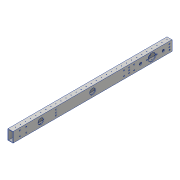
# Autodesk Inventor part: Drive Frame Rail
Saved by Autodesk Inventor 2018 (Build 220112000, 112)
## iProperties
Created: 2018-01-08
Part Number: Drive Frame Rail
Material: Aluminum 6061
Document SubType Name: Modeling
Designer: dsayers
Density: 2.7 g/cm^3
Appearance: Aluminum - Flat
Mass: 735.174 g
Surface Area: 2200.06 cm^2
Volume: 272.287 cm^3
Author: dsayers
Autodesk Inventor part; units mm, degrees
ref_plane "YZ Plane" through (0, 0, 0) normal (1, 0, 0) x (0, 1, 0)
ref_plane "XZ Plane" through (0, 0, 0) normal (0, 1, 0) x (-1, 0, 0)
ref_plane "XY Plane" through (0, 0, 0) normal (0, 0, 1) x (1, 0, 0)
sketch "Sketch1" plane through (0, 0, 0) normal (0, 0, 1) x (1, 0, 0)
  line L0 (0, 0) -> (25.4, 0)
  line L1 (25.4, 0) -> (25.4, 50.8)
  line L2 (25.4, 50.8) -> (0, 50.8)
  line L3 (0, 50.8) -> (0, 0)
  dimension "d0" = 25.4
  dimension "d1" = 50.8
  constraints: 8 end point, 2 parallel, 1 horizontal, 1 perpendicular
  measures "d0" distance of L1.end L2.end
  measures "d1" distance of L0.end L1.end
extrude "Extrusion1" add sketch "Sketch1" along normal blind 800.1
shell "Shell1" thickness 2.54 removed faces 2 at (8.4667, 33.8667, 0) at (8.4667, 33.8667, 800.1)
sketch "Sketch2" plane through (0, 50.8, 0) normal (0, 1, 0) x (1, 0, 0)
  line L0 (25.4, 0) -> (0, 0) projected
  line L1 (0, 0) -> (0, -800.1) projected
  point P0 (12.7, -12.7)
  point P1 (12.7, -38.1)
  point P2 (12.7, -63.5)
  point P3 (12.7, -88.9)
  point P4 (12.7, -114.3)
  point P5 (12.7, -139.7)
  point P6 (12.7, -165.1)
  point P7 (12.7, -190.5)
  point P8 (12.7, -215.9)
  point P9 (12.7, -241.3)
  point P10 (12.7, -266.7)
  point P11 (12.7, -292.1)
  point P12 (12.7, -317.5)
  point P13 (12.7, -342.9)
  point P14 (12.7, -368.3)
  point P15 (12.7, -393.7)
  point P16 (12.7, -419.1)
  point P17 (12.7, -444.5)
  point P18 (12.7, -469.9)
  point P19 (12.7, -495.3)
  point P20 (12.7, -520.7)
  point P21 (12.7, -546.1)
  point P22 (12.7, -571.5)
  point P23 (12.7, -596.9)
  point P24 (12.7, -622.3)
  point P25 (12.7, -647.7)
  point P26 (12.7, -673.1)
  point P27 (12.7, -698.5)
  point P28 (12.7, -723.9)
  point P29 (12.7, -749.3)
  point P30 (12.7, -774.7)
  dimension "d5" = 12.7
  dimension "d6" = 12.7
  dimension "d9" = 25.4
  constraints: 1 vertical, 30 other
  measures "d5" distance from line of L0 point (12.7, -12.7)
  measures "d6" distance from line of L1 point (12.7, -12.7)
  measures "d9" distance of point (12.7, -12.7) point (12.7, -38.1)
hole "Hole1" at (12.7, 50.8, 12.7) at (12.7, 50.8, 38.1) at (12.7, 50.8, 63.5) at (12.7, 50.8, 88.9) at (12.7, 50.8, 114.3) at (12.7, 50.8, 139.7) at (12.7, 50.8, 165.1) at (12.7, 50.8, 190.5) at (12.7, 50.8, 215.9) at (12.7, 50.8, 241.3) at (12.7, 50.8, 266.7) at (12.7, 50.8, 292.1) at (12.7, 50.8, 317.5) at (12.7, 50.8, 342.9) at (12.7, 50.8, 368.3) at (12.7, 50.8, 393.7) at (12.7, 50.8, 419.1) at (12.7, 50.8, 444.5) at (12.7, 50.8, 469.9) at (12.7, 50.8, 495.3) at (12.7, 50.8, 520.7) at (12.7, 50.8, 546.1) at (12.7, 50.8, 571.5) at (12.7, 50.8, 596.9) at (12.7, 50.8, 622.3) at (12.7, 50.8, 647.7) at (12.7, 50.8, 673.1) at (12.7, 50.8, 698.5) at (12.7, 50.8, 723.9) at (12.7, 50.8, 749.3) at (12.7, 50.8, 774.7) direction (0, -1, 0) diameter 2.54 depth 50.8 tip angle 118
sketch "Sketch3" plane through (25.4, 0, 0) normal (1, 0, 0) x (0, 0, -1)
  line L0 (0, 0) -> (0, 50.8) projected
  line L1 (0, 50.8) -> (-800.1, 50.8) projected
  point P0 (-101.6, 25.4)
  dimension "d21" = 101.6
  dimension "d22" = 25.4
  measures "d21" distance from line of L0 point (-101.6, 25.4)
  measures "d22" distance from line of L1 point (-101.6, 25.4)
hole "Hole2" at (25.4, 25.4, 101.6) direction (-1, 0, 0) diameter 38.1 depth 25.4 tip angle 118
sketch "Sketch4" plane through (25.4, 0, 0) normal (1, 0, 0) x (0, 0, -1)
  circle A0 centre (-101.6, 25.4) radius 19.05 projected
  line L0 (0, 0) -> (0, 50.8) projected
  line L1 (0, 50.8) -> (-800.1, 50.8) projected
  line L2 (-800.1, 0) -> (-800.1, 50.8) projected
  line L3 (0, 0) -> (-800.1, 0) projected
  point P0 (0, 0)
  point P1 (-125.4125, 25.4)
  point P2 (-77.7875, 25.4)
  dimension "d30" = 23.8125
  dimension "d31" = 23.8125
  dimension "d32" = 25.4
  dimension "d33" = 25.4
  measures "d30" distance of A0.centre point (-77.788, 25.4)
  measures "d31" distance of point (-125.412, 25.4) A0.centre
  measures "d32" distance from line of point (-77.788, 25.4) L1
  measures "d33" distance from line of L1 point (-125.412, 25.4)
hole "Hole3" at (25.4, 25.4, 125.4125) at (25.4, 25.4, 77.7875) direction (-1, 0, 0) diameter 5.6134 depth 25.4 tip angle 118 clearance for "Flat Head Machine Screw (82)" size "#10" standard "Ansi Unified Screw Threads"
sketch "Sketch5" plane through (25.4, 0, 0) normal (1, 0, 0) x (0, 0, -1)
  circle A0 centre (-44.45, 25.4) radius 8.0391 projected
  circle A1 centre (-158.75, 25.4) radius 9.5885 projected
  point P0 (0, 0)
  point P1 (26.2069, 26.9781)
  constraints: 2 coincident
hole "Hole4" at (25.4, 25.4, 158.75) at (25.4, 25.4, 44.45) at (25.4, 26.9781, -26.2069) direction (-1, 0, 0) diameter 12.7 depth 25.4 tip angle 118
sketch "Sketch6" plane through (0, 0, 0) normal (-1, 0, 0) x (0, 0, 1)
  line L0 (0, 50.8) -> (800.1, 50.8) projected
  line L1 (0, 50.8) -> (0, 0) projected
  line L2 (800.1, 50.8) -> (800.1, 0) projected
  point P0 (400.05, 25.4)
  point P1 (660.4, 25.4)
  dimension "d48" = 25.4
  dimension "d49" = 25.4
  dimension "d50" = 400.05
  dimension "d51" = 400.05
  dimension "d52" = 139.7
  measures "d48" distance from line of L0 point (660.4, 25.4)
  measures "d49" distance from line of L0 point (400.05, 25.4)
  measures "d50" distance from line of L1 point (400.05, 25.4)
  measures "d51" distance from line of L2 point (400.05, 25.4)
  measures "d52" distance from line of L2 point (660.4, 25.4)
hole "Hole5" at (0, 25.4, 400.05) at (0, 25.4, 660.4) direction (1, 0, 0) diameter 28.575 depth 25.4 tip angle 118
sketch "Sketch7" plane through (0, 0, 0) normal (-1, 0, 0) x (0, 0, 1)
  line L0 (723.9, 0) -> (723.9, 609.6)
  line L1 (774.7, 0) -> (774.7, 609.6)
  line L2 (0, 50.8) -> (800.1, 50.8) projected
  line L3 (0, 0) -> (800.1, 0) projected
  point P0 (733.425, 38.1)
  point P1 (765.175, 12.7)
  point P2 (733.425, 12.7)
  point P3 (765.175, 38.1)
  dimension "d60" = 9.525
  dimension "d61" = 9.525
  dimension "d62" = 12.7
  dimension "d63" = 12.7
  dimension "d64" = 12.7
  dimension "d65" = 12.7
  dimension "d66" = 9.525
  dimension "d67" = 9.525
  constraints: 4 end point, 2 vertical, 4 other
  measures "d60" distance from line of L1 point (765.175, 38.1)
  measures "d61" distance from line of L1 point (765.175, 12.7)
  measures "d62" distance from line of L2 point (765.175, 38.1)
  measures "d63" distance from line of L3 point (765.175, 12.7)
  measures "d64" distance from line of L3 point (733.425, 12.7)
  measures "d65" distance from line of L2 point (733.425, 38.1)
  measures "d66" distance from line of L0 point (733.425, 38.1)
  measures "d67" distance from line of L0 point (733.425, 12.7)
hole "Hole6" at (0, 38.1, 733.425) at (0, 12.7, 765.175) at (0, 12.7, 733.425) at (0, 38.1, 765.175) direction (1, 0, 0) diameter 5.6134 depth 25.4 tip angle 118 clearance for "Flat Head Machine Screw (82)" size "#10" standard "Ansi Unified Screw Threads"
sketch "Sketch8" plane through (25.4, 0, 0) normal (1, 0, 0) x (0, 0, -1)
  line L0 (-596.9, 50.8) -> (-596.9, 0) projected
  line L1 (-571.5, 0) -> (-571.5, 50.8) projected
  line L2 (-228.6, 50.8) -> (-228.6, 0) projected
  line L3 (-203.2, 0) -> (-203.2, 50.8) projected
  line L4 (0, 2.54) -> (0, 48.26) projected
  line L5 (-25.4, 50.8) -> (-25.4, 0) projected
  line L6 (0, 0) -> (0, 50.8) projected
  line L7 (0, 0) -> (-800.1, 0) projected
  line L8 (0, 50.8) -> (-800.1, 50.8) projected
  point P0 (-584.2, 38.1)
  point P1 (-584.2, 12.7)
  point P2 (-215.9, 38.1)
  point P3 (-215.9, 12.7)
  point P4 (-12.7, 38.1)
  point P5 (-12.7, 12.7)
  dimension "d75" = 12.7
  dimension "d76" = 12.7
  dimension "d77" = 12.7
  dimension "d78" = 12.7
  dimension "d79" = 12.7
  dimension "d80" = 12.7
  dimension "d81" = 12.7
  dimension "d82" = 12.7
  dimension "d83" = 12.7
  dimension "d84" = 12.7
  dimension "d85" = 12.7
  dimension "d86" = 12.7
  measures "d75" distance from line of point (-12.7, 38.1) L6
  measures "d76" distance from line of L6 point (-12.7, 12.7)
  measures "d77" distance from line of L7 point (-12.7, 12.7)
  measures "d78" distance from line of point (-12.7, 38.1) L8
  measures "d79" distance from line of L3 point (-215.9, 38.1)
  measures "d80" distance from line of L3 point (-215.9, 12.7)
  measures "d81" distance from line of point (-215.9, 12.7) L7
  measures "d82" distance from line of L8 point (-215.9, 38.1)
  measures "d83" distance from line of L1 point (-584.2, 38.1)
  measures "d84" distance from line of L1 point (-584.2, 12.7)
  measures "d85" distance from line of L8 point (-584.2, 38.1)
  measures "d86" distance from line of L7 point (-584.2, 12.7)
hole "Hole7" at (25.4, 38.1, 584.2) at (25.4, 12.7, 584.2) at (25.4, 38.1, 215.9) at (25.4, 12.7, 215.9) at (25.4, 38.1, 12.7) at (25.4, 12.7, 12.7) direction (-1, 0, 0) diameter 5.6134 depth 25.4 tip angle 118 clearance for "Flat Head Machine Screw (82)" size "#10" standard "Ansi Unified Screw Threads"
sketch "Sketch9" plane through (25.4, 0, 0) normal (1, 0, 0) x (0, 0, -1)
  line L0 (0, 2.54) -> (-800.1, 2.54) projected
  circle A0 centre (-12.7, 38.1) radius 2.8067 projected
  circle A1 centre (-215.9, 38.1) radius 2.8067 projected
  circle A2 centre (-584.2, 38.1) radius 2.8067 projected
  circle A3 centre (-584.2, 12.7) radius 2.8067 projected
  circle A4 centre (-215.9, 12.7) radius 2.8067 projected
  circle A5 centre (-12.7, 12.7) radius 2.8067 projected
  circle A6 centre (-733.425, 12.7) radius 2.8067 projected
  circle A7 centre (-733.425, 38.1) radius 2.8067 projected
  circle A8 centre (-765.175, 12.7) radius 2.8067 projected
  circle A9 centre (-765.175, 38.1) radius 2.8067 projected
  circle A10 centre (-400.05, 25.4) radius 14.2875 projected
  circle A11 centre (-660.4, 25.4) radius 14.2875 projected
  circle A12 centre (-44.45, 25.4) radius 6.35 projected
  circle A13 centre (-158.75, 25.4) radius 6.35 projected
  circle A14 centre (-125.4125, 25.4) radius 2.8067 projected
  circle A15 centre (-77.7875, 25.4) radius 2.8067 projected
  circle A16 centre (-101.6, 25.4) radius 19.05 projected
  line L1 (0, 0) -> (0, 50.8) projected
  line L2 (0, 50.8) -> (-800.1, 50.8) projected
  line L3 (-800.1, 0) -> (-800.1, 50.8) projected
  line L4 (0, 0) -> (-800.1, 0) projected
  point P0 (0, 0)
  point P1 (-584.2, 25.4)
  point P2 (-215.9, 25.4)
  point P3 (-12.7, 25.4)
hole "Hole8" at (25.4, 25.4, 584.2) at (25.4, 25.4, 215.9) at (25.4, 25.4, 12.7) direction (-1, 0, 0) diameter 5.6134 depth 25.4 tip angle 118 clearance for "Flat Head Machine Screw (82)" size "#10" standard "Ansi Unified Screw Threads"
sketch "Sketch10" plane through (0, 0, 0) normal (-1, 0, 0) x (0, 0, 1)
  line L0 (0, 50.8) -> (800.1, 50.8) projected
  line L1 (0, 0) -> (800.1, 0) projected
  circle A0 centre (215.9, 12.7) radius 2.8067 projected
  circle A1 centre (215.9, 38.1) radius 2.8067 projected
  point P0 (190.5, 38.1)
  point P1 (190.5, 12.7)
  dimension "d101" = 12.7
  dimension "d102" = 12.7
  dimension "d103" = 25.4
  dimension "d104" = 25.4
  measures "d101" distance from line of L0 point (190.5, 38.1)
  measures "d102" distance from line of L1 point (190.5, 12.7)
  measures "d103" distance of A0.centre point (190.5, 12.7)
  measures "d104" distance of A1.centre point (190.5, 38.1)
hole "Hole9" at (0, 38.1, 190.5) at (0, 12.7, 190.5) direction (1, 0, 0) diameter 5.6134 depth 25.4 tip angle 118 clearance for "Flat Head Machine Screw (82)" size "#10" standard "Ansi Unified Screw Threads"
sketch "Sketch11" plane through (0, 0, 0) normal (-1, 0, 0) x (0, 0, 1)
  circle A0 centre (241.3, 38.1) radius 1.27
  circle A1 centre (241.3, 12.7) radius 1.27
  point P0 (0, 0)
  constraints: 2 centre point, 2 coincident, 4 other
hole "Hole10" at (0, 38.1, 241.3) at (0, 12.7, 241.3) direction (1, 0, 0) diameter 5.6134 depth 25.4 tip angle 118 clearance for "Flat Head Machine Screw (82)" size "#10" standard "Ansi Unified Screw Threads"
equation "\"d50\" = d51"
equation "\"d61\" = d60"
equation "\"d63\" = d62"
equation "\"d64\" = d62"
equation "\"d65\" = d62"
equation "\"d66\" = d61"
equation "\"d67\" = d66"
equation "\"d76\" = d75"
equation "\"d78\" = d77"
equation "\"d79\" = d75"
equation "\"d80\" = d79"
equation "\"d81\" = d77"
equation "\"d82\" = d81"
equation "\"d83\" = d79"
equation "\"d84\" = d83"
equation "\"d85\" = d82"
equation "\"d86\" = d81"
equation "\"d104\" = d103"
body "Solid1"
